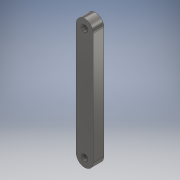
# Autodesk Inventor part: biellette1
Saved by Autodesk Inventor 2017 SP1 (Build 210196100, 196)
## iProperties
Part Number: biellette1
Material: Acier inoxydable
Document SubType Name: Modeling
Designer: Biscuit
Density: 8 g/cm^3
Appearance: Semi-poli
Author: Biscuit
Autodesk Inventor part; units mm, degrees
ref_plane "YZ Plane" through (0, 0, 0) normal (1, 0, 0) x (0, 1, 0)
ref_plane "XZ Plane" through (0, 0, 0) normal (0, 1, 0) x (-1, 0, 0)
ref_plane "XY Plane" through (0, 0, 0) normal (0, 0, 1) x (1, 0, 0)
sketch "Esquisse1" plane through (0, 0, 0) normal (0, 1, 0) x (-1, 0, 0)
  line L0 (0, 0) -> (8, 0)
  line L1 (8, 0) -> (8, -60.5)
  line L2 (8, -60.5) -> (0, -60.5)
  line L3 (0, -60.5) -> (0, 0)
  circle A0 centre (4, -4) radius 1.5
  circle A1 centre (4, -56.5) radius 1.5
  dimension "d1" = 8
  dimension "d2" = 3
  dimension "d3" = 4
  dimension "d4" = 4
  dimension "d5" = 4
  dimension "d6" = 4
  dimension "d7" = 3
  dimension "d11" = 52.5
  constraints: 8 end point, 2 centre point, 2 parallel, 1 horizontal, 1 perpendicular
  measures "d1" distance of L0.start L0.end
  measures "d2" diameter of A0
  measures "d3" distance from line of L1 A0.centre
  measures "d4" distance from line of L0 A0.centre
  measures "d5" distance from line of L3 A1.centre
  measures "d6" distance from line of L2 A1.centre
  measures "d7" diameter of A1
  measures "d11" distance of A1.centre A0.centre
extrude "Extrusion1" add sketch "Esquisse1" along normal blind 5
fillet "Congé1" radius 4 4 edges at (-8, 2.5, 0) (0, 2.5, 0) (0, 2.5, -60.5) (-8, 2.5, -60.5)
equation "\"d3\" = 0.5 * d1"
equation "\"d4\" = d3"
equation "\"d5\" = d3"
equation "\"d6\" = d5"
equation "\"d7\" = d2"
